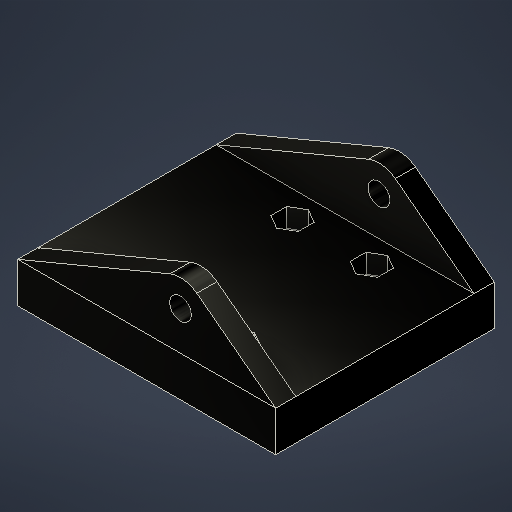
# Autodesk Inventor part: CameraMount
Saved by Autodesk Inventor 2027 (Build 310192000, 192)
## iProperties
Created: 2017-10-01
Part Number: CameraMount
Material: ABS Plastic
Document SubType Name: Modeling
Designer: david
Density: 1.06 g/cm^3
Appearance: Gunmetal
Author: david
Autodesk Inventor part; units mm, degrees
sketch "Sketch1" plane through (0, 0, 0) normal (0, 1, 0) x (-1, 0, 0)
  line L0 (-20.32, 15.1384) -> (-20.32, -15.1384)
  line L1 (-20.32, -15.1384) -> (20.32, -15.1384)
  line L2 (20.32, -15.1384) -> (20.32, 15.1384)
  line L3 (20.32, 15.1384) -> (-20.32, -15.1384) construction
  line L4 (-20.32, 15.1384) -> (20.32, -15.1384) construction
  line L5 (20.32, 15.1384) -> (-20.32, 15.1384)
  point P0 (0, 0)
  dimension "d9" = 30.2768
  dimension "d23" = 40.64
  constraints: 12 end point, 2 midpoint, 2 perpendicular, 1 horizontal, 1 parallel
  measures "d9" distance of L1.end L2.end
  measures "d23" distance of L2.end L0.start
extrude "Extrusion1" add sketch "Sketch1" along normal blind 6.35
sketch "Sketch3" plane through (-20.32, 0, 15.1384) normal (0, 0, 1) x (1, 0, 0)
  point P0 (20.32, 0)
  point P1 (0, 0)
sketch "Sketch4" plane through (20.32, 0, -15.1384) normal (0, 0, -1) x (-1, 0, 0)
  line L0 (0, 0) -> (0, 6.35)
  line L1 (0, 6.35) -> (12.418, 15.828)
  line L2 (40.64, 0) -> (40.64, 6.35)
  line L3 (40.64, 6.35) -> (16.6386, 16.372)
  arc A0 (16.6386, 16.372) -> (12.418, 15.828) centre (14.9993, 12.446) ccw
  line L4 (40.64, 0) -> (0, 0)
  circle A1 centre (14.9993, 12.446) radius 1.7145
  circle A2 centre (14.9993, 12.446) radius 2.4511 projected
  point P0 (20.32, 0)
  dimension "d14" = 3.429
  dimension "d24" = 2.54
  constraints: 10 end point, 2 centre point, 2 coincident, 2 point on circle, 2 tangent, 1 concentric, 1 horizontal, 1 vertical
  measures "d14" diameter of A1
  measures "d24" radial gap between concentric circles of A0 A1
ref_plane "Work Plane5" through (-20.32, 0, 18.3236) normal (0, 0, 1) x (1, 0, 0)
extrude "Extrusion6" add sketch "Sketch4" along normal blind 3.175 contours L0 L1 A0 L3 L2 L4 | A2
sketch "Sketch6" plane through (0, 6.35, 0) normal (0, 1, 0) x (1, 0, 0)
  circle A0 centre (-4.1879, -9.9736) radius 1.05 projected
  circle A1 centre (8.3121, -9.9736) radius 1.05 projected
  circle A2 centre (8.3121, 11.0264) radius 1.05 projected
  circle A3 centre (-4.1879, 11.0264) radius 1.05 projected
  point P0 (0, 0)
extrude "Extrusion7" cut sketch "Sketch6" against normal up to next
ref_plane "Work Plane4" through (-20.32, 0, 18.3236) normal (0, 0, 1) x (1, 0, 0)
sketch "Sketch13" plane through (0, 6.35, 0) normal (0, 1, 0) x (1, 0, 0)
  circle A0 centre (-4.1879, 11.0264) radius 1.05
  line L0 (-2.0289, 9.7799) -> (-4.1879, 8.5334)
  line L1 (-4.1879, 8.5334) -> (-6.3469, 9.7799)
  line L2 (-6.3469, 9.7799) -> (-6.3469, 12.2729)
  line L3 (-6.3469, 12.2729) -> (-4.1879, 13.5194)
  line L4 (-4.1879, 13.5194) -> (-2.0289, 12.2729)
  line L5 (-2.0289, 12.2729) -> (-2.0289, 9.7799)
  circle A1 centre (8.3121, 11.0264) radius 1.05
  line L6 (10.4711, 9.7799) -> (8.3121, 8.5334)
  line L7 (8.3121, 8.5334) -> (6.1531, 9.7799)
  line L8 (6.1531, 9.7799) -> (6.1531, 12.2729)
  line L9 (6.1531, 12.2729) -> (8.3121, 13.5194)
  line L10 (8.3121, 13.5194) -> (10.4711, 12.2729)
  line L11 (10.4711, 12.2729) -> (10.4711, 9.7799)
  circle A2 centre (-4.1879, -9.9736) radius 1.05
  line L12 (-2.0289, -11.2201) -> (-4.1879, -12.4666)
  line L13 (-4.1879, -12.4666) -> (-6.3469, -11.2201)
  line L14 (-6.3469, -11.2201) -> (-6.3469, -8.7271)
  line L15 (-6.3469, -8.7271) -> (-4.1879, -7.4806)
  line L16 (-4.1879, -7.4806) -> (-2.0289, -8.7271)
  line L17 (-2.0289, -8.7271) -> (-2.0289, -11.2201)
  circle A3 centre (8.3121, -9.9736) radius 1.05
  line L18 (10.4711, -11.2201) -> (8.3121, -12.4666)
  line L19 (8.3121, -12.4666) -> (6.1531, -11.2201)
  line L20 (6.1531, -11.2201) -> (6.1531, -8.7271)
  line L21 (6.1531, -8.7271) -> (8.3121, -7.4806)
  line L22 (8.3121, -7.4806) -> (10.4711, -8.7271)
  line L23 (10.4711, -8.7271) -> (10.4711, -11.2201)
  line L24 (-20.32, 15.1384) -> (-20.32, -15.1384) projected
  circle A4 centre (0, 0) radius 1.7967
  constraints: 48 end point, 5 centre point, 5 coincident, 52 other
extrude "Extrusion12" cut sketch "Sketch13" against normal blind 2.9972 contours L0 L1 L2 L3 L4 L5 | L6 L7 L8 L9 L10 L11 | L12 L13 L14 L15 L16 L17 | L18 L19 L20 L21 L22 L23
ref_plane "Work Plane2" through (-20.32, 0, 18.3236) normal (0, 0, 1) x (1, 0, 0)
ref_plane "Work Plane7" through (-20.32, 0, -1.5875) normal (0, 0, 1) x (1, 0, 0)
sketch "Sketch17" plane through (-20.32, 0, 15.1384) normal (0, 0, 1) x (1, 0, 0)
  line L0 (0, 0) -> (0, 6.35) projected
  line L1 (40.64, 6.35) -> (0, 6.35) projected
  line L2 (0, 0) -> (40.64, 0)
  line L3 (40.64, 0) -> (40.64, 6.35)
  line L4 (40.64, 6.35) -> (0, 6.35)
  line L5 (0, 6.35) -> (0, 0)
  point P0 (20.32, 0)
  constraints: 8 end point, 2 parallel, 1 horizontal, 1 perpendicular
extrude "Extrusion16" add sketch "Sketch17" along normal blind 1
ref_plane "Work Plane9" through (-20.32, 0, -1.0877) normal (0, 0, 1) x (1, 0, 0)
mirror "Mirror2" about plane through (-20.32, 0, -1.0877) normal (0, 0, 1) of "Extrusion6"
body "Solid1"
